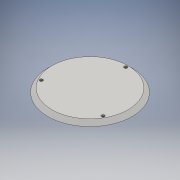
# Autodesk Inventor part: Tampa inferior
Saved by Autodesk Inventor 2016 (Build 200138000, 138)
## iProperties
Created: 2018-11-13
Part Number: Tampa inferior
Material: Genérico
Document SubType Name: Modeling
Designer: thiag
Density: 1 g/cm^3
Appearance: Padrão
Author: thiag
Autodesk Inventor part; units mm, degrees
ref_plane "YZ Plane" through (0, 0, 0) normal (1, 0, 0) x (0, 1, 0)
ref_plane "XZ Plane" through (0, 0, 0) normal (0, 1, 0) x (-1, 0, 0)
ref_plane "XY Plane" through (0, 0, 0) normal (0, 0, 1) x (1, 0, 0)
sketch "Esboço1" plane through (0, 0, 0) normal (0, 0, 1) x (1, 0, 0)
  circle A0 centre (0, 0) radius 26.6
  circle A1 centre (0, 22.6) radius 1
  circle A2 centre (-19.5722, -11.3) radius 1
  circle A3 centre (0, 0) radius 26.6
  circle A4 centre (19.5722, -11.3) radius 1
  circle A5 centre (0, 0) radius 26.6
  dimension "d8" = 360
  constraints: 6 centre point, 3 coincident, 11 other
extrude "Extrusão1" add sketch "Esboço1" along normal blind 2.5
chamfer "Chanfro1" distance 2.5 angle 45 1 edges at (-26.6, 0, 2.5)
chamfer "Chanfro2" distance 1.5 angle 45 3 edges at (18.5722, -11.3, 0) (-20.5722, -11.3, 0) (-1, 22.6, 0)
